Autodesk Fusion 360 part; units mm, degrees
(part 2 of 2)
  constraint tangent A28 A143
  constraint tangent L161 A143
  constraint concentric A143 A144
  constraint parallel L24 L162
  constraint coincident A27 L163.end
  constraint perpendicular L162 L163
  constraint tangent L163 A145
  constraint tangent A27 A145
  constraint perpendicular L4 L164
  constraint coincident A28 L165.end
  constraint perpendicular L5 L165
  constraint tangent L165 A146
  constraint tangent A28 A146
  constraint perpendicular L6 L166
  constraint coincident A25 L167.end
  constraint perpendicular L166 L167
  constraint tangent L167 A147
  constraint tangent A25 A147
  constraint perpendicular L14 L168
  constraint coincident A25 L169.end
  constraint perpendicular L15 L169
  constraint tangent A25 A148
  constraint tangent L169 A148
  constraint perpendicular L16 L170
  constraint coincident A27 L171.end
  constraint perpendicular L170 L171
  constraint tangent L171 A149
  constraint tangent A122 A149
  constraint concentric A149 A150
  constraint concentric A148 A151
  constraint concentric A147 A152
  constraint concentric A146 A153
  constraint concentric A145 A154
  constraint horizontal L172
  constraint vertical L173
  constraint horizontal L174
  constraint vertical L175
  constraint midpoint L173 P11
  constraint coincident L1 P11
  constraint collinear L5 L175
  constraint coincident A156.centre L176.start
  constraint perpendicular L33 L176
  constraint coincident L176.end A157.centre
  constraint horizontal L177
  constraint vertical L178
  constraint horizontal L179
  constraint vertical L180
  constraint coincident L172 L178.end
  constraint horizontal L181
  constraint vertical L182
  constraint horizontal L183
  constraint vertical L184
  constraint coincident L172 L182.end
  constraint horizontal L185
  constraint vertical L186
  constraint horizontal L187
  constraint vertical L188
  constraint coincident L174 L185.start
  constraint coincident L174 L189.start
  constraint perpendicular L174 L189
  constraint coincident L188 L190.end
  constraint perpendicular L188 L190
  constraint coincident L184 L191.start
  constraint perpendicular L184 L191
  constraint coincident L172 L192.end
  constraint perpendicular L172 L192
  constraint tangent L191 A158
  constraint tangent L184 A158
  constraint coincident A158.centre L193.start
  constraint coincident A158 L193.end
  constraint coincident L191 L193.end
  constraint perpendicular L191 L193
  constraint coincident L184 L194.end
  constraint coincident A158 L194.end
  constraint perpendicular L184 L194
  constraint tangent L190 A159
  constraint tangent L188 A159
  constraint coincident A159.centre L195.start
  constraint coincident L190 L195.end
  constraint coincident A159 L195.end
  constraint perpendicular L190 L195
  constraint coincident L188 L196.end
  constraint coincident A159 L196.end
  constraint perpendicular L188 L196
  constraint coincident L197.end A160.centre
  constraint coincident L189.end A160
  constraint coincident L198.end A161.centre
  constraint coincident L187.end A161
  constraint coincident L199.end A162.centre
  constraint coincident L189.start A162
  constraint coincident L200.end A163.centre
  constraint coincident L185.end A163
  constraint coincident L201.end A164.centre
  constraint coincident L186.end A164
  constraint coincident L202.end A165.centre
  constraint coincident L191.end A165
  constraint coincident L203.end A166.centre
  constraint coincident L181.start A166
  constraint coincident L204.end A167.centre
  constraint coincident L181.end A167
  constraint coincident L206.end A168.centre
  constraint coincident L182.end A168
  constraint coincident L205.end A169.centre
  constraint coincident L192.end A169
  constraint coincident L192 L207.start
  constraint coincident A169 L207.start
  constraint coincident A165 L207.end
  constraint coincident L192 L207.end
  constraint coincident L172 L208.start
  constraint coincident A169 L208.start
  constraint coincident A168 L208.end
  constraint coincident L172 L208.end
  constraint coincident A168 L209.start
  constraint coincident L182 L209.start
  constraint coincident A167 L209.end
  constraint coincident L182 L209.end
  constraint coincident A167 L210.start
  constraint coincident L181 L210.start
  constraint coincident A166 L210.end
  constraint coincident L181 L210.end
  constraint coincident L184 L211.start
  constraint coincident A166 L211.start
  constraint coincident L191 L212.end
  constraint coincident A165 L212.end
  constraint coincident L189 L213.start
  constraint coincident A162 L213.start
  constraint coincident A160 L213.end
  constraint coincident L189 L213.end
  constraint coincident L190 L214.start
  constraint coincident A160 L214.start
  constraint coincident L188 L215.end
  constraint coincident A161 L215.end
  constraint coincident L187 L216.start
  constraint coincident A161 L216.start
  constraint coincident A164 L216.end
  constraint coincident L187 L216.end
  constraint coincident L186 L217.start
  constraint coincident A164 L217.start
  constraint coincident L186 L217.end
  constraint coincident A163 L217.end
  constraint coincident L174 L218.start
  constraint coincident A163 L218.start
  constraint coincident L174 L218.end
  constraint coincident A162 L218.end
  constraint horizontal L219
  constraint vertical L220
  constraint horizontal L221
  constraint vertical L222
  constraint perpendicular L187 L223
  constraint coincident P13 L223.end
  constraint coincident P12 L222
  constraint coincident P12 L219
  constraint tangent L222 A182
  constraint tangent L219 A182
  constraint coincident P13 L219
  constraint coincident P13 L220
  constraint tangent L219 A183
  constraint tangent L220 A183
  constraint coincident P14 L222
  constraint coincident P14 L221
  constraint tangent L222 A184
  constraint tangent L221 A184
  constraint tangent L221 A185
  constraint tangent L220 A185
  constraint horizontal L224
  constraint vertical L225
  constraint horizontal L226
  constraint vertical L227
  constraint coincident L228.end A186.centre
  constraint coincident L224.start A186
  constraint coincident L230.end A187.centre
  constraint coincident L226.end A187
  constraint coincident L229.end A188.centre
  constraint coincident L224.end A188
  constraint coincident L231.end A189.centre
  constraint coincident L225.end A189
  constraint coincident L224 L232.start
  constraint coincident A186 L232.start
  constraint coincident L224 L232.end
  constraint coincident A188 L232.end
  constraint coincident L227 L233.start
  constraint coincident A186 L233.start
  constraint coincident A187 L233.end
  constraint coincident L227 L233.end
  constraint coincident L226 L234.start
  constraint coincident A187 L234.start
  constraint coincident L226 L234.end
  constraint coincident A189 L234.end
  constraint coincident L225 L235.start
  constraint coincident A189 L235.start
  constraint coincident A188 L235.end
  constraint coincident L225 L235.end
  constraint horizontal L236
  constraint vertical L237
  constraint horizontal L238
  constraint vertical L239
  constraint perpendicular L181 L240
  constraint coincident L237.end L238.start
  constraint coincident P15 L239
  constraint coincident P15 L236
  constraint tangent L239 A194
  constraint tangent L236 A194
  constraint coincident P16 L236
  constraint coincident P16 L237
  constraint tangent L236 A195
  constraint tangent L237 A195
  constraint coincident P17 L239
  constraint coincident P17 L238
  constraint tangent L239 A196
  constraint tangent L238 A196
  constraint midpoint L239 L241.start
  constraint coincident L237 L241.end
  constraint perpendicular L237 L241
  constraint coincident A197.centre L242.end
  constraint horizontal L242
  measures "d1" diameter of A26
  measures "d2" angle of L1 L2
  measures "d3" angle of L1 L3
  measures "d4" distance of L5.end L6.end
  measures "d5" distance of L4.start L6.end
  measures "d6" diameter of A7
  measures "d7" distance of L5.end L8.end
  measures "d8" angle of L6 L8
  measures "d9" distance of L4.end L9.end
  measures "d10" angle of L4 L9
  measures "d11" diameter of A0
  measures "d12" distance of L13.start L13.end
  measures "d13" distance of L13.start L14.end
  measures "d14" diameter of A9
  measures "d15" diameter of A11
  measures "d16" distance of L14.end L17.end
  measures "d17" angle of L15 L17
  measures "d18" distance of L15.end L18.end
  measures "d19" angle of L15 L18
  measures "d21" distance of L22.start L22.end
  measures "d22" distance of L22.start L23.end
  measures "d23" diameter of A23
  measures "d24" diameter of A21
  measures "d25" distance of L24.end L26.end
  measures "d26" angle of L24 L26
  measures "d27" distance of L23.end L27.end
  measures "d28" angle of L24 L27
  measures "d29" distance of L31.end L32.end
  measures "d30" distance of L7 L32
  measures "d31" distance of L34.start L34.end
  measures "d32" distance of L34.start L36.end
  measures "d34" distance of L32 L35
  measures "d35" distance of L39.start L39.end
  measures "d36" distance of L39.start L41.end
  measures "d37" distance of L35 L42
  measures "d38" distance of L34.start L44.end
  measures "d39" distance of L34.end L45.end
  measures "d40" distance of L36.end L46.end
  measures "d41" distance of L35.end L47.end
  measures "d42" angle of L34 L44
  measures "d43" angle of L34 L45
  measures "d44" angle of L36 L46
  measures "d45" angle of L36 L47
  measures "d46" distance of L39.start L52.end
  measures "d47" distance of L39.end L53.end
  measures "d48" distance of L41.end L54.end
  measures "d49" distance of L40.end L55.end
  measures "d50" angle of L39 L52
  measures "d51" angle of L39 L53
  measures "d52" angle of L41 L54
  measures "d53" angle of L41 L55
  measures "d54" distance of L60.end L61.end
  measures "d55" distance of L13 L61
  measures "d56" distance of L63.end L64.end
  measures "d57" distance of L64.end L65.end
  measures "d58" distance of L61 L65
  measures "d59" distance of L68.end L69.end
  measures "d60" distance of L68.start L68.end
  measures "d61" distance of L65 L68
  measures "d62" distance of L65.end L73.end
  measures "d63" distance of L63.start L74.end
  measures "d64" distance of L63.end L76.end
  measures "d65" distance of L64.end L75.end
  measures "d66" angle of L63 L76
  measures "d67" angle of L65 L75
  measures "d68" angle of L65 L73
  measures "d69" angle of L63 L74
  measures "d70" distance of L70.end L81.end
  measures "d71" distance of L68.start L82.end
  measures "d72" distance of L69.end L83.end
  measures "d73" distance of L68.end L84.end
  measures "d74" angle of L68 L82
  measures "d75" angle of L70 L81
  measures "d76" angle of L70 L83
  measures "d77" angle of L68 L84
  measures "d78" distance of L89.end L90.end
  measures "d79" distance of L22 L90
  measures "d81" distance of L92.end L93.end
  measures "d82" distance of L92.start L92.end
  measures "d83" distance of L90 L94
  measures "d84" distance of L97.end L98.end
  measures "d85" distance of L98.end L99.end
  measures "d86" distance of L94 L97
  measures "d87" distance of L99.end L102.end
  measures "d88" distance of L97.start L103.end
  measures "d89" distance of L98.end L104.end
  measures "d90" distance of L97.end L105.end
  measures "d91" angle of L99 L102
  measures "d92" angle of L99 L104
  measures "d93" angle of L97 L105
  measures "d94" angle of L97 L103
  measures "d95" distance of L94.end L110.end
  measures "d96" distance of L92.start L111.end
  measures "d97" distance of L93.end L112.end
  measures "d98" distance of L92.end L113.end
  measures "d99" angle of L94 L110
  measures "d100" angle of L92 L111
  measures "d101" angle of L94 L112
  measures "d102" angle of L92 L113
  measures "d103" distance of L118.start L120.end
  measures "d104" distance of L0.start L121
  measures "d105" distance of L121 L125
  measures "d106" distance of L122.start L124.end
  measures "d107" distance of L125 L126
  measures "d108" distance of L122 L127.start
  measures "d109" angle of L122 L127
  measures "d110" distance of L124 L128.start
  measures "d111" angle of L124 L128
  measures "d112" distance of L120.end L129.end
  measures "d113" distance of L124.end L130.end
  measures "d114" angle of L120 L129
  measures "d115" angle of L124 L130
  measures "d116" diameter of A103
  measures "d117" distance of L118.start L131.end
  measures "d118" distance of L122.start L132.end
  measures "d119" angle of L118 L131
  measures "d120" angle of L122 L132
  measures "d121" diameter of A106
  measures "d122" diameter of A107
  measures "d123" diameter of A108
  measures "d124" diameter of A109
  measures "d125" diameter of A110
  measures "d131" diameter of A123
  measures "d132" diameter of A124
  measures "d133" diameter of A125
  measures "d134" diameter of A126
  measures "d135" diameter of A127
  measures "d136" diameter of A128
  measures "d137" diameter of A129
  measures "d138" diameter of A130
  measures "d139" diameter of A131
  measures "d140" diameter of A132
  measures "d141" diameter of A133
  measures "d142" diameter of A134
  measures "d143" diameter of A135
  measures "d144" diameter of A136
  measures "d145" diameter of A137
  measures "d146" diameter of A138
  measures "d147" diameter of A139
  measures "d148" diameter of A140
  measures "d149" diameter of A141
  measures "d150" diameter of A142
  measures "d151" distance of L30 L161
  measures "d152" diameter of A143
  measures "d153" diameter of A144
  measures "d154" distance of L28 L163
  measures "d155" diameter of A145
  measures "d156" distance of L12 L165
  measures "d157" diameter of A146
  measures "d158" distance of L10 L167
  measures "d159" diameter of A147
  measures "d160" distance of L21 L169
  measures "d161" diameter of A148
  measures "d162" distance of L19 L171
  measures "d163" diameter of A149
  measures "d164" diameter of A150
  measures "d165" diameter of A151
  measures "d166" diameter of A152
  measures "d167" diameter of A153
  measures "d168" diameter of A154
  measures "d169" distance of L172.start L172.end
  measures "d170" distance of L172.start L174.end
  measures "d171" diameter of A155
  measures "d172" distance of L175 A155.centre
  measures "d173" distance of L174 A155.centre
  measures "d174" diameter of A156
  measures "d175" diameter of A157
  measures "d176" distance of A156.centre L176.end
  measures "d177" distance of L173 L176
  measures "d178" distance of L174 L176.end
  measures "d179" distance of L177.start L179.end
  measures "d180" distance of L177.start L177.end
  measures "d181" distance of L173 L178
  measures "d182" distance of L181.start L183.end
  measures "d183" distance of L181.start L181.end
  measures "d184" distance of L175 L184
  measures "d185" distance of L185.start L185.end
  measures "d186" distance of L185.start L187.end
  measures "d187" distance of L175 L188
  measures "d188" distance of L186 L189
  measures "d189" distance of L189.start L189.end
  measures "d190" distance of L191.end L192.end
  measures "d191" distance of L182 L192
  measures "d192" diameter of A158
  measures "d193" diameter of A159
  measures "d194" distance of L189.end L197.end
  measures "d195" distance of L187.end L198.end
  measures "d196" angle of L190 L197
  measures "d197" angle of L187 L198
  measures "d198" distance of L189.start L199.end
  measures "d199" angle of L174 L199
  measures "d200" distance of L185.end L200.end
  measures "d201" angle of L174 L200
  measures "d202" distance of L186.end L201.end
  measures "d203" angle of L187 L201
  measures "d204" distance of L191.end L202.end
  measures "d205" distance of L181.start L203.end
  measures "d206" distance of L181.end L204.end
  measures "d207" angle of L181 L204
  measures "d208" angle of L181 L203
  measures "d209" angle of L191 L202
  measures "d210" distance of L192.end L205.end
  measures "d211" distance of L182.end L206.end
  measures "d212" angle of L172 L205
  measures "d213" angle of L183 L206
  measures "d214" distance of P12 P13
  measures "d215" distance of P12 P14
  measures "d216" distance of L186.end P13
  measures "d217" radius of A182
  measures "d218" radius of A183
  measures "d219" radius of A184
  measures "d220" radius of A185
  measures "d221" distance of L224.start L224.end
  measures "d222" distance of L224.start L226.end
  measures "d223" distance of L222 L227
  measures "d224" distance of L219 L224
  measures "d225" distance of L224.start L228.end
  measures "d226" distance of L224.end L229.end
  measures "d227" distance of L226.end L230.end
  measures "d228" distance of L225.end L231.end
  measures "d229" angle of L224 L228
  measures "d230" angle of L224 L229
  measures "d231" angle of L226 L231
  measures "d232" angle of L226 L230
  measures "d233" distance of P15 P16
  measures "d234" distance of P15 P17
  measures "d235" distance of L181.end L237.end
  measures "d236" radius of A194
  measures "d237" radius of A195
  measures "d238" radius of A196
  measures "d272" diameter of A197
  measures "d303" distance of L241.end A197.centre
extrude "Extrude1" add sketch "Sketch1" along normal blind 4.8 contours A0 A2 A4 A5 A7 L10 L11 L12 A9 A11 A13 A15 L19 L20 L21 A17 A19 A21 A23 L28 L29 L30 A25 A28 L133 L134 L135 L136 L137 L138 L139 L140 L141 A111 A112 A113 A114 A115 A116 A117 A118 A119 A120 A121 A122 | A144 | A150 | A151 | A152 | A153 | A154 | L219 L220 L221 L222 A182 A183 A184 A185 | L232 L233 L234 L235 A190 A191 A192 A193
sketch "Sketch2" plane through (32, 0, 0) normal (1, 0, 0) x (0, 1, 0)
  line L0 (-16.1787, 0) -> (16.1787, 0)
  line L1 (16.1787, 0) -> (16.1787, 4.8)
  line L2 (16.1787, 4.8) -> (-16.1787, 4.8)
  line L3 (-16.1787, 4.8) -> (-16.1787, 0)
  line L4 (-16.1787, 4.8) -> (16.1787, 0) construction
  circle A0 centre (0, 2.4) radius 1.5
  point P0 (0, 2.4)
  dimension "d128" = 3
  constraint coincident L2.end L3.start
  constraint coincident L0.end L1.start
  constraint midpoint L4 P0
  constraint coincident P0 A0.centre
  measures "d128" diameter of A0
extrude "Extrude2" cut sketch "Sketch2" against normal blind 8 contours A0
thread "Thread1" "ISO Metric profile 3.0 M3x0.5 6H" major diameter 3.086 minor diameter 2.529 pitch 0.5 angle 60 modelled right hand crest width 0.1368 on face at (29.3333, 1.4925, 2.2506) crest through (31.875, 1.2645, 2.4)
sketch "Sketch3" plane through (0, 0, 4.8) normal (0, 0, 1) x (-1, 0, 0)
  arc A0 (-52.8202, -75.7299) -> (-55.718, -76.5064) centre (-54.2691, -76.1181) ccw
  line L0 (-52.8202, -75.7299) -> (-39.1739, -83.6086)
  arc A1 (-38.3975, -86.5064) -> (-39.1739, -83.6086) centre (-38.7857, -85.0575) ccw
  line L1 (-38.3975, -86.5064) -> (-38.6762, -86.9891)
  arc A2 (-41.5739, -87.7655) -> (-38.6762, -86.9891) centre (-40.125, -87.3773) ccw
  line L2 (-41.5739, -87.7655) -> (-55.2202, -79.8868)
  arc A3 (-55.9967, -76.9891) -> (-55.2202, -79.8868) centre (-55.6084, -78.438) ccw
  line L3 (-55.9967, -76.9891) -> (-55.718, -76.5064)
  circle A4 centre (45.4941, -42.5) radius 1.5
  circle A5 centre (64.5, -111.7173) radius 1.5
  arc A6 (94.6728, -10) -> (96.7941, -7.8787) centre (95.7335, -8.9393) ccw
  line L4 (94.6728, -10) -> (94.1155, -10)
  arc A7 (91.9941, -7.8787) -> (94.1155, -10) centre (93.0548, -8.9393) ccw
  line L5 (91.9941, -7.8787) -> (91.9941, 7.8787)
  arc A8 (94.1155, 10) -> (91.9941, 7.8787) centre (93.0548, 8.9393) ccw
  line L6 (94.1155, 10) -> (94.6728, 10)
  arc A9 (96.7941, 7.8787) -> (94.6728, 10) centre (95.7335, 8.9393) ccw
  line L7 (96.7941, 7.8787) -> (96.7941, -7.8787)
  line L8 (48.7941, 89.8787) -> (48.7941, 87.5)
  arc A10 (48.7941, 87.5) -> (50.2941, 86) centre (50.2941, 87.5) ccw
  line L9 (50.2941, 86) -> (55.6728, 86)
  arc A11 (57.7941, 83.8787) -> (55.6728, 86) centre (56.7335, 84.9393) ccw
  line L10 (57.7941, 83.8787) -> (57.7941, 58.1213)
  arc A12 (55.6728, 56) -> (57.7941, 58.1213) centre (56.7335, 57.0607) ccw
  line L11 (55.6728, 56) -> (13.9155, 56)
  arc A13 (11.7941, 58.1213) -> (13.9155, 56) centre (12.8548, 57.0607) ccw
  line L12 (11.7941, 58.1213) -> (11.7941, 89.8787)
  arc A14 (13.9155, 92) -> (11.7941, 89.8787) centre (12.8548, 90.9393) ccw
  line L13 (13.9155, 92) -> (46.6728, 92)
  arc A15 (48.7941, 89.8787) -> (46.6728, 92) centre (47.7335, 90.9393) ccw
  arc A16 (39.8728, -10) -> (41.9941, -7.8787) centre (40.9335, -8.9393) ccw
  line L14 (39.8728, -10) -> (39.3155, -10)
  arc A17 (37.1941, -7.8787) -> (39.3155, -10) centre (38.2548, -8.9393) ccw
  line L15 (37.1941, -7.8787) -> (37.1941, 7.8787)
  arc A18 (39.3155, 10) -> (37.1941, 7.8787) centre (38.2548, 8.9393) ccw
  line L16 (39.3155, 10) -> (39.8728, 10)
  arc A19 (41.9941, 7.8787) -> (39.8728, 10) centre (40.9335, 8.9393) ccw
  line L17 (41.9941, 7.8787) -> (41.9941, -7.8787)
  arc A20 (-11.2762, 39.5309) -> (-14.1739, 40.3073) centre (-12.725, 39.9191) ccw
  line L18 (-11.2762, 39.5309) -> (-10.9975, 39.0482)
  arc A21 (-11.7739, 36.1504) -> (-10.9975, 39.0482) centre (-11.3857, 37.5993) ccw
  line L19 (-11.7739, 36.1504) -> (-25.4202, 28.2717)
  arc A22 (-28.318, 29.0482) -> (-25.4202, 28.2717) centre (-26.8691, 28.66) ccw
  line L20 (-28.318, 29.0482) -> (-28.5967, 29.5309)
  arc A23 (-27.8202, 32.4286) -> (-28.5967, 29.5309) centre (-28.2084, 30.9798) ccw
  line L21 (-27.8202, 32.4286) -> (-14.1739, 40.3073)
  arc A24 (-10.9975, -39.0482) -> (-11.7739, -36.1504) centre (-11.3857, -37.5993) ccw
  line L22 (-10.9975, -39.0482) -> (-11.2762, -39.5309)
  arc A25 (-14.1739, -40.3073) -> (-11.2762, -39.5309) centre (-12.725, -39.9191) ccw
  line L23 (-14.1739, -40.3073) -> (-27.8202, -32.4286)
  arc A26 (-28.5967, -29.5309) -> (-27.8202, -32.4286) centre (-28.2084, -30.9798) ccw
  line L24 (-28.5967, -29.5309) -> (-28.318, -29.0482)
  arc A27 (-25.4202, -28.2717) -> (-28.318, -29.0482) centre (-26.8691, -28.66) ccw
  line L25 (-25.4202, -28.2717) -> (-11.7739, -36.1504)
  circle A28 centre (64.5, 111.7173) radius 1.5
  circle A29 centre (45.4941, 42.5) radius 1.5
  line L26 (55.6728, -86) -> (50.2941, -86)
  arc A30 (50.2941, -86) -> (48.7941, -87.5) centre (50.2941, -87.5) ccw
  line L27 (48.7941, -87.5) -> (48.7941, -89.8787)
  arc A31 (46.6728, -92) -> (48.7941, -89.8787) centre (47.7335, -90.9393) ccw
  line L28 (46.6728, -92) -> (13.9155, -92)
  arc A32 (11.7941, -89.8787) -> (13.9155, -92) centre (12.8548, -90.9393) ccw
  line L29 (11.7941, -89.8787) -> (11.7941, -58.1213)
  arc A33 (13.9155, -56) -> (11.7941, -58.1213) centre (12.8548, -57.0607) ccw
  line L30 (13.9155, -56) -> (55.6728, -56)
  arc A34 (57.7941, -58.1213) -> (55.6728, -56) centre (56.7335, -57.0607) ccw
  line L31 (57.7941, -58.1213) -> (57.7941, -83.8787)
  arc A35 (55.6728, -86) -> (57.7941, -83.8787) centre (56.7335, -84.9393) ccw
  circle A36 centre (-123.5112, 37.2289) radius 1.5
  circle A37 centre (-123.5112, -37.2289) radius 1.5
  arc A38 (-55.2202, 79.8868) -> (-55.9967, 76.9891) centre (-55.6084, 78.438) ccw
  line L32 (-55.2202, 79.8868) -> (-41.5739, 87.7655)
  arc A39 (-38.6762, 86.9891) -> (-41.5739, 87.7655) centre (-40.125, 87.3773) ccw
  line L33 (-38.6762, 86.9891) -> (-38.3975, 86.5064)
  arc A40 (-39.1739, 83.6086) -> (-38.3975, 86.5064) centre (-38.7857, 85.0575) ccw
  line L34 (-39.1739, 83.6086) -> (-52.8202, 75.7299)
  arc A41 (-55.718, 76.5064) -> (-52.8202, 75.7299) centre (-54.2691, 76.1181) ccw
  line L35 (-55.718, 76.5064) -> (-55.9967, 76.9891)
  line L36 (-42.1213, -25.5) -> (-109.5263, -25.5)
  arc A42 (-109.5263, -25.5) -> (-110.7763, -25.8349) centre (-109.5263, -28) ccw
  line L37 (-110.7763, -25.8349) -> (-125.9451, -34.5927)
  arc A43 (-125.9451, -34.5927) -> (-127.0931, -37.4646) centre (-124.6951, -36.7577) ccw
  arc A44 (-127.0931, -37.4646) -> (-89.0244, -98.1371) centre (0, 0) ccw
  arc A45 (-89.0244, -98.1371) -> (-85.1797, -97.5355) centre (-87.3447, -96.2855) ccw
  line L38 (-85.1797, -97.5355) -> (-74.6084, -79.2255)
  arc A46 (-71.7106, -78.449) -> (-74.6084, -79.2255) centre (-73.1595, -78.8372) ccw
  line L39 (-71.7106, -78.449) -> (-32.0836, -101.3277)
  arc A47 (-31.3071, -104.2255) -> (-32.0836, -101.3277) centre (-31.6953, -102.7766) ccw
  line L40 (-31.3071, -104.2255) -> (-41.8784, -122.5355)
  arc A48 (-41.8784, -122.5355) -> (-40.477, -126.166) centre (-39.7133, -123.7855) ccw
  arc A49 (-40.477, -126.166) -> (129.5015, -28.0288) centre (0, 0) ccw
  arc A50 (129.5015, -28.0288) -> (127.0581, -25) centre (127.0581, -27.5) ccw
  line L41 (127.0581, -25) -> (105.9155, -25)
  arc A51 (103.7941, -22.8787) -> (105.9155, -25) centre (104.8548, -23.9393) ccw
  line L42 (103.7941, -22.8787) -> (103.7941, 22.8787)
  arc A52 (105.9155, 25) -> (103.7941, 22.8787) centre (104.8548, 23.9393) ccw
  line L43 (105.9155, 25) -> (127.0581, 25)
  arc A53 (127.0581, 25) -> (129.5015, 28.0288) centre (127.0581, 27.5) ccw
  arc A54 (129.5015, 28.0288) -> (-40.477, 126.166) centre (0, 0) ccw
  arc A55 (-40.477, 126.166) -> (-41.8784, 122.5355) centre (-39.7133, 123.7855) ccw
  line L44 (-41.8784, 122.5355) -> (-31.3071, 104.2255)
  arc A56 (-32.0836, 101.3277) -> (-31.3071, 104.2255) centre (-31.6953, 102.7766) ccw
  line L45 (-32.0836, 101.3277) -> (-71.7106, 78.449)
  arc A57 (-74.6084, 79.2255) -> (-71.7106, 78.449) centre (-73.1595, 78.8372) ccw
  line L46 (-74.6084, 79.2255) -> (-85.1797, 97.5355)
  arc A58 (-85.1797, 97.5355) -> (-89.0244, 98.1371) centre (-87.3447, 96.2855) ccw
  arc A59 (-89.0244, 98.1371) -> (-127.0931, 37.4646) centre (0, 0) ccw
  arc A60 (-127.0931, 37.4646) -> (-125.9451, 34.5927) centre (-124.6951, 36.7577) ccw
  line L47 (-125.9451, 34.5927) -> (-110.7763, 25.8349)
  arc A61 (-110.7763, 25.8349) -> (-109.5263, 25.5) centre (-109.5263, 28) ccw
  line L48 (-109.5263, 25.5) -> (-42.1213, 25.5)
  arc A62 (-40, 23.3787) -> (-42.1213, 25.5) centre (-41.0607, 24.4393) ccw
  line L49 (-40, 23.3787) -> (-40, 20.8)
  arc A63 (-40, 20.8) -> (-37.5, 18.3) centre (-37.5, 20.8) ccw
  line L50 (-37.5, 18.3) -> (-34.1213, 18.3)
  arc A64 (-32, 16.1787) -> (-34.1213, 18.3) centre (-33.0607, 17.2393) ccw
  line L51 (-32, 16.1787) -> (-32, -16.1787)
  arc A65 (-34.1213, -18.3) -> (-32, -16.1787) centre (-33.0607, -17.2393) ccw
  line L52 (-34.1213, -18.3) -> (-37.5, -18.3)
  arc A66 (-37.5, -18.3) -> (-40, -20.8) centre (-37.5, -20.8) ccw
  line L53 (-40, -20.8) -> (-40, -23.3787)
  arc A67 (-42.1213, -25.5) -> (-40, -23.3787) centre (-41.0607, -24.4393) ccw
  line L54 (41.8941, -111.4) -> (15.4941, -111.4)
  line L55 (11.7941, -107.7) -> (11.7941, -100.7)
  line L56 (15.4941, -97) -> (41.8941, -97)
  line L57 (45.5941, -100.7) -> (45.5941, -107.7)
  line L58 (11.7941, -92) -> (11.7941, -97) construction
  arc A68 (41.8941, -111.4) -> (45.5941, -107.7) centre (41.8941, -107.7) ccw
  arc A69 (45.5941, -100.7) -> (41.8941, -97) centre (41.8941, -100.7) ccw
  arc A70 (11.7941, -107.7) -> (15.4941, -111.4) centre (15.4941, -107.7) ccw
  arc A71 (15.4941, -97) -> (11.7941, -100.7) centre (15.4941, -100.7) ccw
  line L59 (43.7441, -109.75) -> (13.6441, -109.75) construction
  line L60 (13.6441, -109.75) -> (13.6441, -98.65) construction
  line L61 (13.6441, -98.65) -> (43.7441, -98.65) construction
  line L62 (43.7441, -98.65) -> (43.7441, -109.75) construction
  line L63 (43.7441, -109.75) -> (42.6835, -108.6893) construction
  line L64 (13.6441, -109.75) -> (14.7048, -108.6893) construction
  line L65 (43.7441, -98.65) -> (42.6835, -99.7107) construction
  line L66 (13.6441, -98.65) -> (14.7048, -99.7107) construction
  arc A72 (41.6228, -109.75) -> (43.7441, -107.6287) centre (42.6835, -108.6893) ccw
  arc A73 (43.7441, -107.6287) -> (41.6228, -109.75) centre (42.6835, -108.6893) ccw construction
  arc A74 (43.7441, -100.7713) -> (41.6228, -98.65) centre (42.6835, -99.7107) ccw
  arc A75 (41.6228, -98.65) -> (43.7441, -100.7713) centre (42.6835, -99.7107) ccw construction
  arc A76 (15.7655, -98.65) -> (13.6441, -100.7713) centre (14.7048, -99.7107) ccw
  arc A77 (13.6441, -100.7713) -> (15.7655, -98.65) centre (14.7048, -99.7107) ccw construction
  arc A78 (13.6441, -107.6287) -> (15.7655, -109.75) centre (14.7048, -108.6893) ccw
  arc A79 (15.7655, -109.75) -> (13.6441, -107.6287) centre (14.7048, -108.6893) ccw construction
  line L67 (43.7441, -107.6287) -> (43.7441, -100.7713)
  line L68 (41.6228, -98.65) -> (15.7655, -98.65)
  line L69 (13.6441, -100.7713) -> (13.6441, -107.6287)
  line L70 (15.7655, -109.75) -> (41.6228, -109.75)
  circle A80 centre (1.7941, -104.2) radius 5.5
  circle A81 centre (1.7941, -104.2) radius 6.1
  point P0 (45.5941, -111.4)
  point P1 (11.7941, -111.4)
  point P2 (45.5941, -97)
  point P3 (11.7941, -92)
  dimension "d239" = 33.8
  dimension "d240" = 14.4
  dimension "d241" = 5
  dimension "d242" = 3.7
  dimension "d243" = 3.7
  dimension "d244" = 3.7
  dimension "d245" = 3.7
  dimension "d246" = 30.1
  dimension "d247" = 11.1
  dimension "d248" = 1.85
  dimension "d249" = 1.65
  dimension "d250" = 1.5
  dimension "d251" = 1.5
  dimension "d252" = 1.5
  dimension "d253" = 1.5
  dimension "d254" = 45
  dimension "d255" = 45
  dimension "d256" = 45
  dimension "d257" = 45
  dimension "d274" = 12.2
  constraint horizontal L54
  constraint vertical L55
  constraint horizontal L56
  constraint vertical L57
  constraint coincident P3 L58.start
  constraint vertical L58
  constraint coincident P0 L57
  constraint coincident P0 L54
  constraint tangent L57 A68
  constraint tangent L54 A68
  constraint coincident P2 L57
  constraint coincident P2 L56
  constraint tangent L57 A69
  constraint tangent L56 A69
  constraint coincident P1 L54
  constraint coincident P1 L55
  constraint tangent L54 A70
  constraint tangent L55 A70
  constraint coincident L58.end L56
  constraint coincident L58.end L55
  constraint tangent L56 A71
  constraint tangent L55 A71
  constraint horizontal L59
  constraint vertical L60
  constraint horizontal L61
  constraint vertical L62
  constraint coincident L63.end A72.centre
  constraint coincident L59.start A72
  constraint coincident L64.end A78.centre
  constraint coincident L59.end A78
  constraint coincident L66.end A76.centre
  constraint coincident L60.end A76
  constraint coincident L65.end A74.centre
  constraint coincident L61.end A74
  constraint coincident L62 A72.end
  constraint coincident L59 A72.start
  constraint concentric A72 A73
  constraint coincident L61 A74.end
  constraint coincident L62 A74.start
  constraint concentric A74 A75
  constraint coincident L60 A76.end
  constraint coincident L61 A76.start
  constraint concentric A76 A77
  constraint coincident L59 A78.end
  constraint coincident L60 A78.start
  constraint concentric A78 A79
  constraint concentric A80 A81
  measures "d239" distance of P0 P1
  measures "d240" distance of P0 P2
  measures "d241" distance of L58.end P3
  measures "d242" radius of A68
  measures "d243" radius of A69
  measures "d244" radius of A70
  measures "d245" radius of A71
  measures "d246" distance of L59.start L59.end
  measures "d247" distance of L59.start L61.end
  measures "d248" distance of L57 L62
  measures "d249" distance of L54 L59
  measures "d250" distance of L59.start L63.end
  measures "d251" distance of L59.end L64.end
  measures "d252" distance of L61.end L65.end
  measures "d253" distance of L60.end L66.end
  measures "d254" angle of L59 L63
  measures "d255" angle of L59 L64
  measures "d256" angle of L61 L65
  measures "d257" angle of L61 L66
  measures "d274" diameter of A81
extrude "Extrude3" cut sketch "Sketch1" along normal through all contours L232 L233 L234 L235 A190 A191 A192 A193
extrude "Extrude4" cut sketch "Sketch3" against normal through all contours A72 A74 A76 A78 L67 L68 L69 L70
extrude "Extrude5" cut sketch "Sketch3" against normal blind 2.3 contours L54 L55 L56 L57 A68 A69 A70 A71
sketch "Sketch4" plane through (0, 0, 4.8) normal (0, 0, 1) x (-1, 0, 0)
  line L0 (43.7441, 100.7713) -> (43.7441, 107.6287)
  line L1 (41.6228, 98.65) -> (15.7655, 98.65)
  line L2 (41.8941, 97) -> (15.4941, 97)
  line L3 (11.7941, 100.7) -> (11.7941, 107.7)
  line L4 (15.4941, 111.4) -> (41.8941, 111.4)
  line L5 (45.5941, 107.7) -> (45.5941, 100.7)
  arc A0 (41.8941, 97) -> (45.5941, 100.7) centre (41.8941, 100.7) ccw
  arc A1 (11.7941, 100.7) -> (15.4941, 97) centre (15.4941, 100.7) ccw
  arc A2 (45.5941, 107.7) -> (41.8941, 111.4) centre (41.8941, 107.7) ccw
  arc A3 (15.4941, 111.4) -> (11.7941, 107.7) centre (15.4941, 107.7) ccw
  point P0 (45.5941, 97)
  point P1 (11.7941, 97)
  point P2 (45.5941, 111.4)
  dimension "d262" = 33.8
  dimension "d263" = 14.4
  dimension "d264" = 1.85
  dimension "d265" = 1.65
  dimension "d266" = 3.7
  dimension "d267" = 3.7
  dimension "d268" = 3.7
  dimension "d269" = 3.7
  constraint horizontal L2
  constraint vertical L3
  constraint horizontal L4
  constraint vertical L5
  constraint coincident P0 L5
  constraint coincident P0 L2
  constraint tangent L5 A0
  constraint tangent L2 A0
  constraint coincident P1 L2
  constraint coincident P1 L3
  constraint tangent L2 A1
  constraint tangent L3 A1
  constraint coincident P2 L5
  constraint coincident P2 L4
  constraint tangent L5 A2
  constraint tangent L4 A2
  constraint tangent L4 A3
  constraint tangent L3 A3
  measures "d262" distance of P0 P1
  measures "d263" distance of P0 P2
  measures "d264" distance of L0 L5
  measures "d265" distance of L1 L2
  measures "d266" radius of A0
  measures "d267" radius of A1
  measures "d268" radius of A2
  measures "d269" radius of A3
extrude "Extrude6" cut sketch "Sketch4" against normal blind 2.3
extrude "Extrude7" cut sketch "Sketch3" against normal blind 2 contours A81
sketch "Sketch5" plane through (0, 0, 4.8) normal (0, 0, 1) x (-1, 0, 0)
  circle A0 centre (1.7941, -104.2) radius 6.1
  line L0 (15.4941, 111.4) -> (41.8941, 111.4)
  arc A1 (45.5941, 107.7) -> (41.8941, 111.4) centre (41.8941, 107.7) ccw
  line L1 (45.5941, 107.7) -> (45.5941, 100.7)
  arc A2 (41.8941, 97) -> (45.5941, 100.7) centre (41.8941, 100.7) ccw
  line L2 (41.8941, 97) -> (15.4941, 97)
  arc A3 (11.7941, 100.7) -> (15.4941, 97) centre (15.4941, 100.7) ccw
  line L3 (11.7941, 100.7) -> (11.7941, 107.7)
  arc A4 (15.4941, 111.4) -> (11.7941, 107.7) centre (15.4941, 107.7) ccw
  line L4 (15.4941, -97) -> (41.8941, -97)
  arc A5 (45.5941, -100.7) -> (41.8941, -97) centre (41.8941, -100.7) ccw
  line L5 (45.5941, -100.7) -> (45.5941, -107.7)
  arc A6 (41.8941, -111.4) -> (45.5941, -107.7) centre (41.8941, -107.7) ccw
  line L6 (41.8941, -111.4) -> (15.4941, -111.4)
  arc A7 (11.7941, -107.7) -> (15.4941, -111.4) centre (15.4941, -107.7) ccw
  line L7 (11.7941, -107.7) -> (11.7941, -100.7)
  arc A8 (15.4941, -97) -> (11.7941, -100.7) centre (15.4941, -100.7) ccw
  arc A9 (-52.8202, -75.7299) -> (-55.718, -76.5064) centre (-54.2691, -76.1181) ccw
  line L8 (-52.8202, -75.7299) -> (-39.1739, -83.6086)
  arc A10 (-38.3975, -86.5064) -> (-39.1739, -83.6086) centre (-38.7857, -85.0575) ccw
  line L9 (-38.3975, -86.5064) -> (-38.6762, -86.9891)
  arc A11 (-41.5739, -87.7655) -> (-38.6762, -86.9891) centre (-40.125, -87.3773) ccw
  line L10 (-41.5739, -87.7655) -> (-55.2202, -79.8868)
  arc A12 (-55.9967, -76.9891) -> (-55.2202, -79.8868) centre (-55.6084, -78.438) ccw
  line L11 (-55.9967, -76.9891) -> (-55.718, -76.5064)
  line L12 (55.6728, -86) -> (50.2941, -86)
  arc A13 (50.2941, -86) -> (48.7941, -87.5) centre (50.2941, -87.5) ccw
  line L13 (48.7941, -87.5) -> (48.7941, -89.8787)
  arc A14 (46.6728, -92) -> (48.7941, -89.8787) centre (47.7335, -90.9393) ccw
  line L14 (46.6728, -92) -> (13.9155, -92)
  arc A15 (11.7941, -89.8787) -> (13.9155, -92) centre (12.8548, -90.9393) ccw
  line L15 (11.7941, -89.8787) -> (11.7941, -58.1213)
  arc A16 (13.9155, -56) -> (11.7941, -58.1213) centre (12.8548, -57.0607) ccw
  line L16 (13.9155, -56) -> (55.6728, -56)
  line L17 (57.7941, -58.1213) -> (57.7941, -83.8787)
  arc A17 (55.6728, -86) -> (57.7941, -83.8787) centre (56.7335, -84.9393) ccw
  arc A18 (-11.2762, 39.5309) -> (-14.1739, 40.3073) centre (-12.725, 39.9191) ccw
  line L18 (-11.2762, 39.5309) -> (-10.9975, 39.0482)
  arc A19 (-11.7739, 36.1504) -> (-10.9975, 39.0482) centre (-11.3857, 37.5993) ccw
  line L19 (-11.7739, 36.1504) -> (-25.4202, 28.2717)
  arc A20 (-28.318, 29.0482) -> (-25.4202, 28.2717) centre (-26.8691, 28.66) ccw
  line L20 (-28.318, 29.0482) -> (-28.5967, 29.5309)
  arc A21 (-27.8202, 32.4286) -> (-28.5967, 29.5309) centre (-28.2084, 30.9798) ccw
  line L21 (-27.8202, 32.4286) -> (-14.1739, 40.3073)
  arc A22 (-10.9975, -39.0482) -> (-11.7739, -36.1504) centre (-11.3857, -37.5993) ccw
  line L22 (-10.9975, -39.0482) -> (-11.2762, -39.5309)
  arc A23 (-14.1739, -40.3073) -> (-11.2762, -39.5309) centre (-12.725, -39.9191) ccw
  line L23 (-14.1739, -40.3073) -> (-27.8202, -32.4286)
  arc A24 (-28.5967, -29.5309) -> (-27.8202, -32.4286) centre (-28.2084, -30.9798) ccw
  line L24 (-28.5967, -29.5309) -> (-28.318, -29.0482)
  arc A25 (-25.4202, -28.2717) -> (-28.318, -29.0482) centre (-26.8691, -28.66) ccw
  line L25 (-25.4202, -28.2717) -> (-11.7739, -36.1504)
  circle A26 centre (45.4941, -42.5) radius 1.5
  circle A27 centre (-123.5112, -37.2289) radius 1.5
  arc A28 (-55.2202, 79.8868) -> (-55.9967, 76.9891) centre (-55.6084, 78.438) ccw
  line L26 (-55.2202, 79.8868) -> (-41.5739, 87.7655)
  arc A29 (-38.6762, 86.9891) -> (-41.5739, 87.7655) centre (-40.125, 87.3773) ccw
  line L27 (-38.6762, 86.9891) -> (-38.3975, 86.5064)
  arc A30 (-39.1739, 83.6086) -> (-38.3975, 86.5064) centre (-38.7857, 85.0575) ccw
  line L28 (-39.1739, 83.6086) -> (-52.8202, 75.7299)
  arc A31 (-55.718, 76.5064) -> (-52.8202, 75.7299) centre (-54.2691, 76.1181) ccw
  line L29 (-55.718, 76.5064) -> (-55.9967, 76.9891)
  circle A32 centre (64.5, -111.7173) radius 1.5
  arc A33 (94.6728, -10) -> (96.7941, -7.8787) centre (95.7335, -8.9393) ccw
  line L30 (94.6728, -10) -> (94.1155, -10)
  arc A34 (91.9941, -7.8787) -> (94.1155, -10) centre (93.0548, -8.9393) ccw
  line L31 (91.9941, -7.8787) -> (91.9941, 7.8787)
  arc A35 (94.1155, 10) -> (91.9941, 7.8787) centre (93.0548, 8.9393) ccw
  line L32 (94.1155, 10) -> (94.6728, 10)
  arc A36 (96.7941, 7.8787) -> (94.6728, 10) centre (95.7335, 8.9393) ccw
  line L33 (96.7941, 7.8787) -> (96.7941, -7.8787)
  circle A37 centre (45.4941, 42.5) radius 1.5
  arc A38 (39.8728, -10) -> (41.9941, -7.8787) centre (40.9335, -8.9393) ccw
  line L34 (39.8728, -10) -> (39.3155, -10)
  arc A39 (37.1941, -7.8787) -> (39.3155, -10) centre (38.2548, -8.9393) ccw
  line L35 (37.1941, -7.8787) -> (37.1941, 7.8787)
  arc A40 (39.3155, 10) -> (37.1941, 7.8787) centre (38.2548, 8.9393) ccw
  line L36 (39.3155, 10) -> (39.8728, 10)
  arc A41 (41.9941, 7.8787) -> (39.8728, 10) centre (40.9335, 8.9393) ccw
  line L37 (41.9941, 7.8787) -> (41.9941, -7.8787)
  circle A42 centre (64.5, 111.7173) radius 1.5
  circle A43 centre (-123.5112, 37.2289) radius 1.5
  line L38 (48.7941, 89.8787) -> (48.7941, 87.5)
  arc A44 (48.7941, 87.5) -> (50.2941, 86) centre (50.2941, 87.5) ccw
  line L39 (50.2941, 86) -> (55.6728, 86)
  arc A45 (57.7941, 83.8787) -> (55.6728, 86) centre (56.7335, 84.9393) ccw
  line L40 (57.7941, 83.8787) -> (57.7941, 58.1213)
  line L41 (55.6728, 56) -> (13.9155, 56)
  arc A46 (11.7941, 58.1213) -> (13.9155, 56) centre (12.8548, 57.0607) ccw
  line L42 (11.7941, 58.1213) -> (11.7941, 89.8787)
  arc A47 (13.9155, 92) -> (11.7941, 89.8787) centre (12.8548, 90.9393) ccw
  line L43 (13.9155, 92) -> (46.6728, 92)
  arc A48 (48.7941, 89.8787) -> (46.6728, 92) centre (47.7335, 90.9393) ccw
  line L44 (-42.1213, -25.5) -> (-109.5263, -25.5)
  arc A49 (-109.5263, -25.5) -> (-110.7763, -25.8349) centre (-109.5263, -28) ccw
  line L45 (-110.7763, -25.8349) -> (-125.9451, -34.5927)
  arc A50 (-125.9451, -34.5927) -> (-127.0931, -37.4646) centre (-124.6951, -36.7577) ccw
  arc A51 (-127.0931, -37.4646) -> (-89.0244, -98.1371) centre (0, 0) ccw
  arc A52 (-89.0244, -98.1371) -> (-85.1797, -97.5355) centre (-87.3447, -96.2855) ccw
  line L46 (-85.1797, -97.5355) -> (-74.6084, -79.2255)
  arc A53 (-71.7106, -78.449) -> (-74.6084, -79.2255) centre (-73.1595, -78.8372) ccw
  line L47 (-71.7106, -78.449) -> (-32.0836, -101.3277)
  arc A54 (-31.3071, -104.2255) -> (-32.0836, -101.3277) centre (-31.6953, -102.7766) ccw
  line L48 (-31.3071, -104.2255) -> (-41.8784, -122.5355)
  arc A55 (-41.8784, -122.5355) -> (-40.477, -126.166) centre (-39.7133, -123.7855) ccw
  arc A56 (-40.477, -126.166) -> (129.5015, -28.0288) centre (0, 0) ccw
  arc A57 (129.5015, -28.0288) -> (127.0581, -25) centre (127.0581, -27.5) ccw
  line L49 (127.0581, -25) -> (105.9155, -25)
  arc A58 (103.7941, -22.8787) -> (105.9155, -25) centre (104.8548, -23.9393) ccw
  line L50 (103.7941, -22.8787) -> (103.7941, 22.8787)
  arc A59 (105.9155, 25) -> (103.7941, 22.8787) centre (104.8548, 23.9393) ccw
  line L51 (105.9155, 25) -> (127.0581, 25)
  arc A60 (127.0581, 25) -> (129.5015, 28.0288) centre (127.0581, 27.5) ccw
  arc A61 (129.5015, 28.0288) -> (-40.477, 126.166) centre (0, 0) ccw
  arc A62 (-40.477, 126.166) -> (-41.8784, 122.5355) centre (-39.7133, 123.7855) ccw
  line L52 (-41.8784, 122.5355) -> (-31.3071, 104.2255)
  arc A63 (-32.0836, 101.3277) -> (-31.3071, 104.2255) centre (-31.6953, 102.7766) ccw
  line L53 (-32.0836, 101.3277) -> (-71.7106, 78.449)
  arc A64 (-74.6084, 79.2255) -> (-71.7106, 78.449) centre (-73.1595, 78.8372) ccw
  line L54 (-74.6084, 79.2255) -> (-85.1797, 97.5355)
  arc A65 (-85.1797, 97.5355) -> (-89.0244, 98.1371) centre (-87.3447, 96.2855) ccw
  arc A66 (-89.0244, 98.1371) -> (-127.0931, 37.4646) centre (0, 0) ccw
  arc A67 (-127.0931, 37.4646) -> (-125.9451, 34.5927) centre (-124.6951, 36.7577) ccw
  line L55 (-125.9451, 34.5927) -> (-110.7763, 25.8349)
  arc A68 (-110.7763, 25.8349) -> (-109.5263, 25.5) centre (-109.5263, 28) ccw
  line L56 (-109.5263, 25.5) -> (-42.1213, 25.5)
  arc A69 (-40, 23.3787) -> (-42.1213, 25.5) centre (-41.0607, 24.4393) ccw
  line L57 (-40, 23.3787) -> (-40, 20.8)
  arc A70 (-40, 20.8) -> (-37.5, 18.3) centre (-37.5, 20.8) ccw
  line L58 (-37.5, 18.3) -> (-34.1213, 18.3)
  arc A71 (-32, 16.1787) -> (-34.1213, 18.3) centre (-33.0607, 17.2393) ccw
  line L59 (-32, 16.1787) -> (-32, -16.1787)
  arc A72 (-34.1213, -18.3) -> (-32, -16.1787) centre (-33.0607, -17.2393) ccw
  line L60 (-34.1213, -18.3) -> (-37.5, -18.3)
  arc A73 (-37.5, -18.3) -> (-40, -20.8) centre (-37.5, -20.8) ccw
  line L61 (-40, -20.8) -> (-40, -23.3787)
  arc A74 (-42.1213, -25.5) -> (-40, -23.3787) centre (-41.0607, -24.4393) ccw
  line L62 (103.7941, 56) -> (103.7941, -56)
  line L63 (103.7941, -56) -> (-12.8059, -56)
  line L64 (-12.8059, 56) -> (103.7941, 56)
  line L65 (57.7941, 58.1213) -> (57.7941, 83.8787)
  line L66 (57.7941, -58.1213) -> (57.7941, -83.8787)
  line L67 (103.7941, 60) -> (57.7941, 60) construction
  line L68 (57.7941, 60) -> (57.7941, 64.8) construction
  line L69 (57.7941, 64.8) -> (103.7941, 64.8) construction
  line L70 (103.7941, 64.8) -> (103.7941, 60) construction
  line L71 (103.7941, -60) -> (57.7941, -60) construction
  line L72 (57.7941, -60) -> (57.7941, -64.8) construction
  line L73 (57.7941, -64.8) -> (103.7941, -64.8) construction
  line L74 (103.7941, -64.8) -> (103.7941, -60) construction
  line L75 (0, 0) -> (132.5, 0) construction
  line L76 (80.7941, -60) -> (80.7941, 60) construction
  line L77 (90.7941, -64.8) -> (90.7941, -60) construction
  line L78 (70.7941, -64.8) -> (70.7941, -60) construction
  line L79 (90.7941, -60) -> (103.7941, -64.8) construction
  line L80 (70.7941, -60) -> (57.7941, -64.8) construction
  line L81 (90.7941, 60) -> (90.7941, 64.8) construction
  line L82 (90.7941, 60) -> (103.7941, 64.8) construction
  line L83 (70.7941, 64.8) -> (70.7941, 60) construction
  line L84 (70.7941, 60) -> (57.7941, 64.8) construction
  circle A75 centre (97.2941, 62.4) radius 1.5
  circle A76 centre (64.2941, 62.4) radius 1.5
  circle A77 centre (64.2941, -62.4) radius 1.5
  circle A78 centre (97.2941, -62.4) radius 1.5
  point P0 (80.7941, 0)
  point P1 (97.2941, -62.4)
  point P2 (64.2941, -62.4)
  point P3 (97.2941, 62.4)
  point P4 (64.2941, 62.4)
  dimension "d290" = 46
  dimension "d291" = 4.8
  dimension "d292" = 46
  dimension "d293" = 4.8
  dimension "d294" = 120
  dimension "d295" = 13
  dimension "d296" = 13
  dimension "d297" = 13
  dimension "d298" = 13
  dimension "d299" = 3
  dimension "d300" = 3
  dimension "d301" = 3
  dimension "d302" = 3
  constraint horizontal L67
  constraint vertical L68
  constraint horizontal L69
  constraint vertical L70
  constraint coincident L65 L68.end
  constraint horizontal L71
  constraint vertical L72
  constraint horizontal L73
  constraint vertical L74
  constraint coincident L66 L72.end
  constraint midpoint L71 L76.start
  constraint midpoint L67 L76.end
  constraint midpoint L76 P0
  constraint coincident L75 P0
  constraint coincident L73 L77.start
  constraint coincident L71 L77.end
  constraint perpendicular L71 L77
  constraint coincident L73 L78.start
  constraint coincident L71 L78.end
  constraint perpendicular L71 L78
  constraint coincident L67 L81.start
  constraint coincident L69 L81.end
  constraint perpendicular L69 L81
  constraint coincident L69 L83.start
  constraint coincident L67 L83.end
  constraint perpendicular L67 L83
  constraint midpoint L79 P1
  constraint midpoint L80 P2
  constraint midpoint L82 P3
  constraint midpoint L84 P4
  constraint coincident P3 A75.centre
  constraint coincident P4 A76.centre
  constraint coincident P2 A77.centre
  constraint coincident P1 A78.centre
  measures "d290" distance of L68.end L69.end
  measures "d291" distance of L67.start L69.end
  measures "d292" distance of L72.end L73.end
  measures "d293" distance of L71.start L73.end
  measures "d294" distance of L67 L71
  measures "d295" distance of L68 L83
  measures "d296" distance of L70 L81
  measures "d297" distance of L74 L77
  measures "d298" distance of L72 L78
  measures "d299" diameter of A75
  measures "d300" diameter of A76
  measures "d301" diameter of A77
  measures "d302" diameter of A78
extrude "Extrude8" cut sketch "Sketch5" against normal through all contours A75 | A76 | A77 | A78
